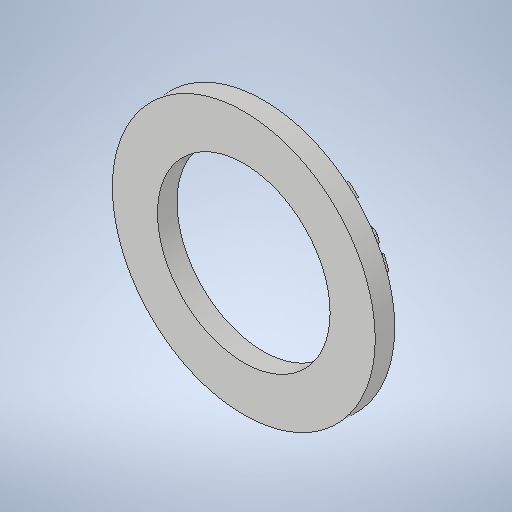
# Autodesk Inventor part: Fixierplatte_Innenring35mm
Saved by Autodesk Inventor 2025 (Build 290162000, 162)
## iProperties
Created: 2020-01-21
Part Number: Fixierplatte_Innenring35mm
Material: Generisch
Document SubType Name: Modeling
Designer: maxse
Density: 1 g/cm^3
Appearance: Vorgabe
Author: maxse
Autodesk Inventor part; units mm, degrees
(part 1 of 2)
ref_plane "YZ Plane" through (0, 0, 0) normal (1, 0, 0) x (0, 1, 0)
ref_plane "XZ Plane" through (0, 0, 0) normal (0, 1, 0) x (-1, 0, 0)
ref_plane "XY Plane" through (0, 0, 0) normal (0, 0, 1) x (1, 0, 0)
sketch "Skizze1" plane through (0, 0, 0) normal (0, 1, 0) x (-1, 0, 0)
  circle A0 centre (0, 0) radius 17.665
  circle A1 centre (0, 0) radius 26.9
  dimension "d0" = 35.33
  dimension "d1" = 53.8
  constraints: 2 centre point, 2 coincident
  measures "d0" diameter of A0
  measures "d1" diameter of A1
extrude "Extrusion1" add sketch "Skizze1" along normal blind 4
sketch "Skizze2" plane through (0, 4, 0) normal (0, 1, 0) x (1, 0, 0)
  circle A0 centre (0, 0) radius 19.096
  spline S0 degree 2 poles (20.5196, -9.7896) (20.1844, -9.6564) (19.6974, -9.2143) (19.5643, -8.9347) knots 0 0 0 1 2 2 2
  spline S1 degree 2 poles (19.5643, -8.9347) (19.4313, -8.6551) (19.4185, -7.9742) (19.5621, -7.6127) knots 0 0 0 1 2 2 2
  spline S2 degree 2 poles (19.5621, -7.6127) (19.6938, -7.2814) (20.098, -6.6921) (20.309, -6.5012) knots 0 0 0 1 2 2 2
  line L0 (20.309, -6.5012) -> (20.968, -6.7631)
  line L1 (20.968, -6.7631) -> (20.95, -6.8083)
  spline S3 degree 2 poles (20.95, -6.8083) (20.8689, -6.8589) (20.6271, -7.0724) (20.5025, -7.2103) knots 0 0 0 1 2 2 2
  spline S4 degree 2 poles (20.5025, -7.2103) (20.3652, -7.3694) (20.1724, -7.646) (20.0961, -7.838) knots 0 0 0 1 2 2 2
  spline S5 degree 2 poles (20.0961, -7.838) (20.0213, -8.0263) (20.0162, -8.4341) (20.1121, -8.6205) knots 0 0 0 1 2 2 2
  spline S6 degree 2 poles (20.1121, -8.6205) (20.2051, -8.7926) (20.5262, -9.0597) (20.7747, -9.1585) knots 0 0 0 1 2 2 2
  spline S7 degree 2 poles (20.7747, -9.1585) (21.0232, -9.2572) (21.3934, -9.2474) (21.5497, -9.1613) knots 0 0 0 1 2 2 2
  spline S8 degree 2 poles (21.5497, -9.1613) (21.7188, -9.0759) (21.9723, -8.7232) (22.0666, -8.4859) knots 0 0 0 1 2 2 2
  spline S9 degree 2 poles (22.0666, -8.4859) (22.1684, -8.2299) (22.2913, -7.6901) (22.3188, -7.5223) knots 0 0 0 1 2 2 2
  line L2 (22.3188, -7.5223) -> (24.7136, -8.474)
  line L3 (24.7136, -8.474) -> (23.7005, -11.0232)
  line L4 (23.7005, -11.0232) -> (23.1545, -10.8062)
  line L5 (23.1545, -10.8062) -> (23.9297, -8.8557)
  line L6 (23.9297, -8.8557) -> (22.6908, -8.3634)
  spline S10 degree 2 poles (22.6908, -8.3634) (22.661, -8.4824) (22.5855, -8.7052) (22.5496, -8.7956) knots 0 0 0 1 2 2 2
  spline S11 degree 2 poles (22.5496, -8.7956) (22.4074, -9.1533) (22.0947, -9.6002) (21.8317, -9.7573) knots 0 0 0 1 2 2 2
  spline S12 degree 2 poles (21.8317, -9.7573) (21.5672, -9.9182) (20.9413, -9.9572) (20.5196, -9.7896) knots 0 0 0 1 2 2 2
  spline S13 degree 2 poles (21.8528, -13.3779) (21.9489, -13.223) (22.0634, -12.8696) (22.0968, -12.6852) knots 0 0 0 1 2 2 2
  spline S14 degree 2 poles (22.0968, -12.6852) (22.1238, -12.5112) (22.126, -12.2312) (22.1201, -12.1178) knots 0 0 0 1 2 2 2
  line L7 (22.1201, -12.1178) -> (22.1414, -12.0834)
  line L8 (22.1414, -12.0834) -> (22.7438, -12.4574)
  spline S15 degree 2 poles (22.7438, -12.4574) (22.7282, -12.7053) (22.4946, -13.4425) (22.3172, -13.7283) knots 0 0 0 1 2 2 2
  spline S16 degree 2 poles (22.3172, -13.7283) (22.1377, -14.0174) (21.7535, -14.375) (21.5206, -14.4736) knots 0 0 0 1 2 2 2
  spline S17 degree 2 poles (21.5206, -14.4736) (21.2709, -14.5762) (20.7622, -14.5274) (20.5006, -14.365) knots 0 0 0 1 2 2 2
  spline S18 degree 2 poles (20.5006, -14.365) (20.1495, -14.147) (19.9058, -13.3565) (20.0378, -12.9902) knots 0 0 0 1 2 2 2
  line L9 (20.0378, -12.9902) -> (19.9965, -12.9646)
  spline S19 degree 2 poles (19.9965, -12.9646) (19.8856, -13.0817) (19.5715, -13.3111) (19.3664, -13.365) knots 0 0 0 1 2 2 2
  spline S20 degree 2 poles (19.3664, -13.365) (19.1647, -13.421) (18.6765, -13.3468) (18.3977, -13.1737) knots 0 0 0 1 2 2 2
  spline S21 degree 2 poles (18.3977, -13.1737) (18.112, -12.9963) (17.7485, -12.4987) (17.6737, -12.2043) knots 0 0 0 1 2 2 2
  spline S22 degree 2 poles (17.6737, -12.2043) (17.5964, -11.8987) (17.7237, -11.2481) (17.9311, -10.9142) knots 0 0 0 1 2 2 2
  spline S23 degree 2 poles (17.9311, -10.9142) (18.1298, -10.5941) (18.6737, -10.0638) (18.913, -9.9166) knots 0 0 0 1 2 2 2
  line L10 (18.913, -9.9166) -> (19.5154, -10.2906)
  line L11 (19.5154, -10.2906) -> (19.4897, -10.3319)
  spline S24 degree 2 poles (19.4897, -10.3319) (19.2478, -10.4297) (18.6306, -10.886) (18.4447, -11.1854) knots 0 0 0 1 2 2 2
  spline S25 degree 2 poles (18.4447, -11.1854) (18.3357, -11.361) (18.2278, -11.7805) (18.2825, -11.9766) knots 0 0 0 1 2 2 2
  spline S26 degree 2 poles (18.2825, -11.9766) (18.3393, -12.1693) (18.5675, -12.4779) (18.7981, -12.6211) knots 0 0 0 1 2 2 2
  spline S27 degree 2 poles (18.7981, -12.6211) (19.0287, -12.7643) (19.4116, -12.816) (19.5724, -12.7489) knots 0 0 0 1 2 2 2
  spline S28 degree 2 poles (19.5724, -12.7489) (19.7333, -12.6819) (20.0017, -12.3955) (20.1214, -12.2027) knots 0 0 0 1 2 2 2
  line L12 (20.1214, -12.2027) -> (20.271, -11.9617)
  line L13 (20.271, -11.9617) -> (20.7426, -12.2546)
  line L14 (20.7426, -12.2546) -> (20.6251, -12.4439)
  spline S29 degree 2 poles (20.6251, -12.4439) (20.3878, -12.826) (20.4535, -13.5345) (20.8012, -13.7503) knots 0 0 0 1 2 2 2
  spline S30 degree 2 poles (20.8012, -13.7503) (20.9629, -13.8508) (21.2705, -13.8701) (21.4014, -13.813) knots 0 0 0 1 2 2 2
  spline S31 degree 2 poles (21.4014, -13.813) (21.5399, -13.7512) (21.7609, -13.5259) (21.8528, -13.3779) knots 0 0 0 1 2 2 2
  line L15 (15.967, -13.7933) -> (16.4799, -13.1765)
  line L16 (16.4799, -13.1765) -> (17.2152, -13.7878)
  line L17 (17.2152, -13.7878) -> (16.7022, -14.4047)
  line L18 (16.7022, -14.4047) -> (15.967, -13.7933)
  spline S32 degree 2 poles (14.1579, -17.7888) (13.915, -17.5223) (13.6708, -16.9115) (13.6737, -16.6019) knots 0 0 0 1 2 2 2
  spline S33 degree 2 poles (13.6737, -16.6019) (13.6765, -16.2923) (13.9633, -15.6746) (14.2508, -15.4125) knots 0 0 0 1 2 2 2
  spline S34 degree 2 poles (14.2508, -15.4125) (14.5143, -15.1723) (15.1358, -14.8197) (15.4091, -14.7405) knots 0 0 0 1 2 2 2
  line L19 (15.4091, -14.7405) -> (15.8867, -15.2646)
  line L20 (15.8867, -15.2646) -> (15.8508, -15.2973)
  spline S35 degree 2 poles (15.8508, -15.2973) (15.7557, -15.3073) (15.4448, -15.3933) (15.2724, -15.4627) knots 0 0 0 1 2 2 2
  spline S36 degree 2 poles (15.2724, -15.4627) (15.0793, -15.5456) (14.7848, -15.7097) (14.6321, -15.8489) knots 0 0 0 1 2 2 2
  spline S37 degree 2 poles (14.6321, -15.8489) (14.4824, -15.9854) (14.2991, -16.3498) (14.3038, -16.5594) knots 0 0 0 1 2 2 2
  spline S38 degree 2 poles (14.3038, -16.5594) (14.3119, -16.7548) (14.4836, -17.1356) (14.6637, -17.3333) knots 0 0 0 1 2 2 2
  spline S39 degree 2 poles (14.6637, -17.3333) (14.8439, -17.5309) (15.181, -17.6842) (15.3592, -17.6752) knots 0 0 0 1 2 2 2
  spline S40 degree 2 poles (15.3592, -17.6752) (15.5486, -17.6725) (15.931, -17.4665) (16.1197, -17.2946) knots 0 0 0 1 2 2 2
  spline S41 degree 2 poles (16.1197, -17.2946) (16.3233, -17.109) (16.6703, -16.6776) (16.7685, -16.5387) knots 0 0 0 1 2 2 2
  line L21 (16.7685, -16.5387) -> (18.5044, -18.4433)
  line L22 (18.5044, -18.4433) -> (16.4771, -20.2912)
  line L23 (16.4771, -20.2912) -> (16.0813, -19.8569)
  line L24 (16.0813, -19.8569) -> (17.6325, -18.4431)
  line L25 (17.6325, -18.4431) -> (16.7345, -17.4579)
  spline S42 degree 2 poles (16.7345, -17.4579) (16.6556, -17.5517) (16.4901, -17.719) (16.4182, -17.7845) knots 0 0 0 1 2 2 2
  spline S43 degree 2 poles (16.4182, -17.7845) (16.1337, -18.0438) (15.6568, -18.3085) (15.3516, -18.3346) knots 0 0 0 1 2 2 2
  spline S44 degree 2 poles (15.3516, -18.3346) (15.0434, -18.3633) (14.4636, -18.1242) (14.1579, -17.7888) knots 0 0 0 1 2 2 2
  line L26 (8.7906, -19.2639) -> (9.8592, -21.1546)
  spline S45 degree 2 poles (9.8592, -21.1546) (9.9868, -21.3804) (10.2394, -21.745) (10.3556, -21.8189) knots 0 0 0 1 2 2 2
  spline S46 degree 2 poles (10.3556, -21.8189) (10.4779, -21.9034) (10.7568, -21.8947) (10.9438, -21.789) knots 0 0 0 1 2 2 2
  spline S47 degree 2 poles (10.9438, -21.789) (11.1131, -21.6933) (11.3835, -21.2659) (11.4765, -20.9527) knots 0 0 0 1 2 2 2
  spline S48 degree 2 poles (11.4765, -20.9527) (11.445, -20.9053) (11.3602, -20.7717) (11.3084, -20.68) knots 0 0 0 1 2 2 2
  line L27 (11.3084, -20.68) -> (10.0923, -18.5283)
  line L28 (10.0923, -18.5283) -> (10.6426, -18.2173)
  line L29 (10.6426, -18.2173) -> (11.7111, -20.108)
  spline S49 degree 2 poles (11.7111, -20.108) (11.8387, -20.3338) (12.0913, -20.6983) (12.2076, -20.7722) knots 0 0 0 1 2 2 2
  spline S50 degree 2 poles (12.2076, -20.7722) (12.3298, -20.8567) (12.6088, -20.848) (12.7957, -20.7424) knots 0 0 0 1 2 2 2
  spline S51 degree 2 poles (12.7957, -20.7424) (12.9721, -20.6427) (13.238, -20.1992) (13.3238, -19.9226) knots 0 0 0 1 2 2 2
  line L30 (13.3238, -19.9226) -> (11.9442, -17.4816)
  line L31 (11.9442, -17.4816) -> (12.4945, -17.1706)
  line L32 (12.4945, -17.1706) -> (14.3406, -20.4371)
  line L33 (14.3406, -20.4371) -> (13.7903, -20.7481)
  line L34 (13.7903, -20.7481) -> (13.5869, -20.3883)
  spline S52 degree 2 poles (13.5869, -20.3883) (13.4934, -20.7251) (13.2036, -21.2006) (12.9497, -21.3442) knots 0 0 0 1 2 2 2
  spline S53 degree 2 poles (12.9497, -21.3442) (12.6604, -21.5076) (12.0629, -21.4963) (11.777, -21.2622) knots 0 0 0 1 2 2 2
  spline S54 degree 2 poles (11.777, -21.2622) (11.6841, -21.6824) (11.3729, -22.2353) (11.0977, -22.3908) knots 0 0 0 1 2 2 2
  spline S55 degree 2 poles (11.0977, -22.3908) (10.8861, -22.5104) (10.4666, -22.5753) (10.2559, -22.4989) knots 0 0 0 1 2 2 2
  spline S56 degree 2 poles (10.2559, -22.4989) (10.0417, -22.4245) (9.6458, -22.0618) (9.4565, -21.7267) knots 0 0 0 1 2 2 2
  line L35 (9.4565, -21.7267) -> (8.2403, -19.5749)
  line L36 (8.2403, -19.5749) -> (8.7906, -19.2639)
  line L37 (3.2919, -20.9174) -> (3.8132, -23.0257)
  spline S57 degree 2 poles (3.8132, -23.0257) (3.8755, -23.2774) (4.0208, -23.6964) (4.1129, -23.7989) knots 0 0 0 1 2 2 2
  spline S58 degree 2 poles (4.1129, -23.7989) (4.2079, -23.9131) (4.479, -23.9797) (4.6875, -23.9281) knots 0 0 0 1 2 2 2
  spline S59 degree 2 poles (4.6875, -23.9281) (4.8763, -23.8814) (5.2516, -23.5424) (5.4252, -23.2657) knots 0 0 0 1 2 2 2
  spline S60 degree 2 poles (5.4252, -23.2657) (5.4077, -23.2116) (5.3619, -23.0601) (5.3366, -22.9579) knots 0 0 0 1 2 2 2
  line L38 (5.3366, -22.9579) -> (4.7433, -20.5585)
  line L39 (4.7433, -20.5585) -> (5.3569, -20.4068)
  line L40 (5.3569, -20.4068) -> (5.8782, -22.5151)
  spline S61 degree 2 poles (5.8782, -22.5151) (5.9405, -22.7668) (6.0858, -23.1858) (6.178, -23.2883) knots 0 0 0 1 2 2 2
  spline S62 degree 2 poles (6.178, -23.2883) (6.273, -23.4025) (6.544, -23.469) (6.7525, -23.4175) knots 0 0 0 1 2 2 2
  spline S63 degree 2 poles (6.7525, -23.4175) (6.9492, -23.3689) (7.3245, -23.0131) (7.4814, -22.7698) knots 0 0 0 1 2 2 2
  line L41 (7.4814, -22.7698) -> (6.8083, -20.0479)
  line L42 (6.8083, -20.0479) -> (7.422, -19.8962)
  line L43 (7.422, -19.8962) -> (8.3226, -23.5385)
  line L44 (8.3226, -23.5385) -> (7.709, -23.6902)
  line L45 (7.709, -23.6902) -> (7.6098, -23.289)
  spline S64 degree 2 poles (7.6098, -23.289) (7.4292, -23.5883) (7.0223, -23.9685) (6.7391, -24.0385) knots 0 0 0 1 2 2 2
  spline S65 degree 2 poles (6.7391, -24.0385) (6.4166, -24.1183) (5.8441, -23.9468) (5.6316, -23.6446) knots 0 0 0 1 2 2 2
  spline S66 degree 2 poles (5.6316, -23.6446) (5.4292, -24.0244) (4.9809, -24.4733) (4.6741, -24.5492) knots 0 0 0 1 2 2 2
  spline S67 degree 2 poles (4.6741, -24.5492) (4.4381, -24.6075) (4.0166, -24.5573) (3.8342, -24.4271) knots 0 0 0 1 2 2 2
  spline S68 degree 2 poles (3.8342, -24.4271) (3.6478, -24.2979) (3.364, -23.8422) (3.2716, -23.4685) knots 0 0 0 1 2 2 2
  line L46 (3.2716, -23.4685) -> (2.6783, -21.0691)
  line L47 (2.6783, -21.0691) -> (3.2919, -20.9174)
  spline S69 degree 2 poles (-1.4876, -20.975) (-0.9736, -21.0007) (-0.4242, -21.6163) (-0.4558, -22.2516) knots 0 0 0 1 2 2 2
  line L48 (-0.4558, -22.2516) -> (-0.5593, -24.3277)
  line L49 (-0.5593, -24.3277) -> (-0.1344, -24.3488)
  line L50 (-0.1344, -24.3488) -> (-0.1604, -24.8709)
  line L51 (-0.1604, -24.8709) -> (-0.5853, -24.8497)
  line L52 (-0.5853, -24.8497) -> (-0.639, -25.9262)
  line L53 (-0.639, -25.9262) -> (-1.2703, -25.8947)
  line L54 (-1.2703, -25.8947) -> (-1.2166, -24.8182)
  line L55 (-1.2166, -24.8182) -> (-2.3781, -24.7604)
  line L56 (-2.3781, -24.7604) -> (-2.3521, -24.2383)
  line L57 (-2.3521, -24.2383) -> (-1.1906, -24.2962)
  line L58 (-1.1906, -24.2962) -> (-1.1017, -22.5115)
  spline S70 degree 2 poles (-1.1017, -22.5115) (-1.0876, -22.2283) (-1.0923, -21.9157) (-1.1544, -21.7787) knots 0 0 0 1 2 2 2
  spline S71 degree 2 poles (-1.1544, -21.7787) (-1.2052, -21.6585) (-1.4543, -21.5284) (-1.6728, -21.5175) knots 0 0 0 1 2 2 2
  spline S72 degree 2 poles (-1.6728, -21.5175) (-1.8266, -21.5099) (-2.1186, -21.5886) (-2.1847, -21.6137) knots 0 0 0 1 2 2 2
  line L59 (-2.1847, -21.6137) -> (-2.2212, -21.6119)
  line L60 (-2.2212, -21.6119) -> (-2.1929, -21.0454)
  spline S73 degree 2 poles (-2.1929, -21.0454) (-2.0124, -21.0057) (-1.6454, -20.9672) (-1.4876, -20.975) knots 0 0 0 1 2 2 2
  spline S74 degree 2 poles (-6.0395, -22.2271) (-5.8581, -21.2965) (-4.7656, -20.4568) (-4.018, -20.6025) knots 0 0 0 1 2 2 2
  spline S75 degree 2 poles (-4.018, -20.6025) (-3.2504, -20.7521) (-2.5754, -21.9694) (-2.7506, -22.8682) knots 0 0 0 1 2 2 2
  spline S76 degree 2 poles (-2.7506, -22.8682) (-2.9304, -23.7909) (-4.0364, -24.6362) (-4.7761, -24.492) knots 0 0 0 1 2 2 2
  spline S77 degree 2 poles (-4.7761, -24.492) (-5.5238, -24.3463) (-6.2202, -23.1538) (-6.0395, -22.2271) knots 0 0 0 1 2 2 2
  spline S78 degree 2 poles (-5.3992, -22.3519) (-5.5388, -23.0678) (-5.1535, -23.8653) (-4.6722, -23.9591) knots 0 0 0 1 2 2 2
  spline S79 degree 2 poles (-4.6722, -23.9591) (-4.191, -24.0529) (-3.5304, -23.4593) (-3.3909, -22.7434) knots 0 0 0 1 2 2 2
  spline S80 degree 2 poles (-3.3909, -22.7434) (-3.2552, -22.0474) (-3.6406, -21.2292) (-4.1218, -21.1354) knots 0 0 0 1 2 2 2
  spline S81 degree 2 poles (-4.1218, -21.1354) (-4.5991, -21.0424) (-5.2613, -21.644) (-5.3992, -22.3519) knots 0 0 0 1 2 2 2
  spline S82 degree 2 poles (-11.4852, -22.9042) (-11.3227, -22.9869) (-10.9609, -23.0712) (-10.7744, -23.0889) knots 0 0 0 1 2 2 2
  spline S83 degree 2 poles (-10.7744, -23.0889) (-10.5987, -23.1011) (-10.3195, -23.0796) (-10.207, -23.0641) knots 0 0 0 1 2 2 2
  line L61 (-10.207, -23.0641) -> (-10.1709, -23.0825)
  line L62 (-10.1709, -23.0825) -> (-10.4928, -23.7144)
  spline S84 degree 2 poles (-10.4928, -23.7144) (-10.7411, -23.7197) (-11.4954, -23.5492) (-11.7951, -23.3966) knots 0 0 0 1 2 2 2
  spline S85 degree 2 poles (-11.7951, -23.3966) (-12.0984, -23.2421) (-12.4872, -22.8894) (-12.6051, -22.6657) knots 0 0 0 1 2 2 2
  spline S86 degree 2 poles (-12.6051, -22.6657) (-12.7283, -22.4255) (-12.7227, -21.9146) (-12.5829, -21.6402) knots 0 0 0 1 2 2 2
  spline S87 degree 2 poles (-12.5829, -21.6402) (-12.3953, -21.2719) (-11.6283, -20.9623) (-11.2521, -21.063) knots 0 0 0 1 2 2 2
  line L63 (-11.2521, -21.063) -> (-11.2301, -21.0197)
  spline S88 degree 2 poles (-11.2301, -21.0197) (-11.3562, -20.9191) (-11.6113, -20.6254) (-11.6823, -20.4256) knots 0 0 0 1 2 2 2
  spline S89 degree 2 poles (-11.6823, -20.4256) (-11.7551, -20.2293) (-11.7224, -19.7367) (-11.5735, -19.4442) knots 0 0 0 1 2 2 2
  spline S90 degree 2 poles (-11.5735, -19.4442) (-11.4208, -19.1445) (-10.9557, -18.7403) (-10.6686, -18.641) knots 0 0 0 1 2 2 2
  spline S91 degree 2 poles (-10.6686, -18.641) (-10.3707, -18.5381) (-9.7116, -18.6101) (-9.3614, -18.7885) knots 0 0 0 1 2 2 2
  spline S92 degree 2 poles (-9.3614, -18.7885) (-9.0256, -18.9595) (-8.4513, -19.4567) (-8.2845, -19.6826) knots 0 0 0 1 2 2 2
  line L64 (-8.2845, -19.6826) -> (-8.6063, -20.3145)
  line L65 (-8.6063, -20.3145) -> (-8.6496, -20.2924)
  spline S93 degree 2 poles (-8.6496, -20.2924) (-8.7675, -20.0596) (-9.2742, -19.4832) (-9.5883, -19.3232) knots 0 0 0 1 2 2 2
  spline S94 degree 2 poles (-9.5883, -19.3232) (-9.7724, -19.2294) (-10.1996, -19.1573) (-10.3904, -19.2284) knots 0 0 0 1 2 2 2
  spline S95 degree 2 poles (-10.3904, -19.2284) (-10.5775, -19.3013) (-10.8658, -19.5546) (-10.989, -19.7965) knots 0 0 0 1 2 2 2
  spline S96 degree 2 poles (-10.989, -19.7965) (-11.1122, -20.0384) (-11.1314, -20.4242) (-11.051, -20.5789) knots 0 0 0 1 2 2 2
  spline S97 degree 2 poles (-11.051, -20.5789) (-10.9706, -20.7335) (-10.6626, -20.9768) (-10.4604, -21.0798) knots 0 0 0 1 2 2 2
  line L66 (-10.4604, -21.0798) -> (-10.2077, -21.2085)
  line L67 (-10.2077, -21.2085) -> (-10.4596, -21.7032)
  line L68 (-10.4596, -21.7032) -> (-10.6582, -21.602)
  spline S98 degree 2 poles (-10.6582, -21.602) (-11.0589, -21.3979) (-11.7593, -21.5231) (-11.9451, -21.8878) knots 0 0 0 1 2 2 2
  spline S99 degree 2 poles (-11.9451, -21.8878) (-12.0315, -22.0575) (-12.0248, -22.3656) (-11.9569, -22.4911) knots 0 0 0 1 2 2 2
  spline S100 degree 2 poles (-11.9569, -22.4911) (-11.8836, -22.6239) (-11.6404, -22.8251) (-11.4852, -22.9042) knots 0 0 0 1 2 2 2
  spline S101 degree 2 poles (-14.9124, -17.1612) (-14.6946, -16.8738) (-14.1385, -16.5225) (-13.8336, -16.4689) knots 0 0 0 1 2 2 2
  spline S102 degree 2 poles (-13.8336, -16.4689) (-13.5286, -16.4153) (-12.869, -16.5848) (-12.559, -16.8197) knots 0 0 0 1 2 2 2
  spline S103 degree 2 poles (-12.559, -16.8197) (-12.2748, -17.0351) (-11.8148, -17.582) (-11.6872, -17.8362) knots 0 0 0 1 2 2 2
  line L69 (-11.6872, -17.8362) -> (-12.1155, -18.4014)
  line L70 (-12.1155, -18.4014) -> (-12.1543, -18.372)
  spline S104 degree 2 poles (-12.1543, -18.372) (-12.1814, -18.2803) (-12.3225, -17.9903) (-12.4222, -17.8334) knots 0 0 0 1 2 2 2
  spline S105 degree 2 poles (-12.4222, -17.8334) (-12.5389, -17.6586) (-12.7539, -17.399) (-12.9186, -17.2741) knots 0 0 0 1 2 2 2
  spline S106 degree 2 poles (-12.9186, -17.2741) (-13.0801, -17.1518) (-13.4718, -17.038) (-13.677, -17.0807) knots 0 0 0 1 2 2 2
  spline S107 degree 2 poles (-13.677, -17.0807) (-13.8677, -17.1243) (-14.2108, -17.3625) (-14.3724, -17.5756) knots 0 0 0 1 2 2 2
  spline S108 degree 2 poles (-14.3724, -17.5756) (-14.5339, -17.7887) (-14.6232, -18.1481) (-14.5819, -18.3217) knots 0 0 0 1 2 2 2
  spline S109 degree 2 poles (-14.5819, -18.3217) (-14.5448, -18.5075) (-14.2726, -18.846) (-14.0691, -19.0002) knots 0 0 0 1 2 2 2
  spline S110 degree 2 poles (-14.0691, -19.0002) (-13.8495, -19.1666) (-13.3622, -19.4292) (-13.2078, -19.5004) knots 0 0 0 1 2 2 2
  line L71 (-13.2078, -19.5004) -> (-14.7643, -21.5542)
  line L72 (-14.7643, -21.5542) -> (-16.9505, -19.8974)
  line L73 (-16.9505, -19.8974) -> (-16.5956, -19.4292)
  line L74 (-16.5956, -19.4292) -> (-14.9229, -20.6969)
  line L75 (-14.9229, -20.6969) -> (-14.1177, -19.6345)
  spline S111 degree 2 poles (-14.1177, -19.6345) (-14.2244, -19.5739) (-14.419, -19.4417) (-14.4965, -19.383) knots 0 0 0 1 2 2 2
  spline S112 degree 2 poles (-14.4965, -19.383) (-14.8033, -19.1505) (-15.1504, -18.7297) (-15.2316, -18.4344) knots 0 0 0 1 2 2 2
  spline S113 degree 2 poles (-15.2316, -18.4344) (-15.316, -18.1365) (-15.1865, -17.5229) (-14.9124, -17.1612) knots 0 0 0 1 2 2 2
  line L76 (-17.3405, -12.1524) -> (-19.0049, -13.5475)
  spline S114 degree 2 poles (-19.0049, -13.5475) (-19.2037, -13.7141) (-19.5161, -14.0288) (-19.5677, -14.1566) knots 0 0 0 1 2 2 2
  spline S115 degree 2 poles (-19.5677, -14.1566) (-19.6285, -14.2922) (-19.5691, -14.5649) (-19.4311, -14.7295) knots 0 0 0 1 2 2 2
  spline S116 degree 2 poles (-19.4311, -14.7295) (-19.3062, -14.8785) (-18.8367, -15.0666) (-18.5118, -15.1009) knots 0 0 0 1 2 2 2
  spline S117 degree 2 poles (-18.5118, -15.1009) (-18.471, -15.0614) (-18.3551, -14.9537) (-18.2743, -14.886) knots 0 0 0 1 2 2 2
  line L77 (-18.2743, -14.886) -> (-16.3801, -13.2983)
  line L78 (-16.3801, -13.2983) -> (-15.974, -13.7827)
  line L79 (-15.974, -13.7827) -> (-17.6385, -15.1778)
  spline S118 degree 2 poles (-17.6385, -15.1778) (-17.8372, -15.3444) (-18.1497, -15.6591) (-18.2012, -15.7869) knots 0 0 0 1 2 2 2
  spline S119 degree 2 poles (-18.2012, -15.7869) (-18.262, -15.9225) (-18.2026, -16.1952) (-18.0647, -16.3598) knots 0 0 0 1 2 2 2
  spline S120 degree 2 poles (-18.0647, -16.3598) (-17.9345, -16.5151) (-17.45, -16.6958) (-17.1625, -16.7297) knots 0 0 0 1 2 2 2
  line L80 (-17.1625, -16.7297) -> (-15.0136, -14.9286)
  line L81 (-15.0136, -14.9286) -> (-14.6076, -15.413)
  line L82 (-14.6076, -15.413) -> (-17.4831, -17.8232)
  line L83 (-17.4831, -17.8232) -> (-17.8891, -17.3388)
  line L84 (-17.8891, -17.3388) -> (-17.5724, -17.0733)
  spline S121 degree 2 poles (-17.5724, -17.0733) (-17.9206, -17.0426) (-18.441, -16.8444) (-18.6284, -16.6208) knots 0 0 0 1 2 2 2
  spline S122 degree 2 poles (-18.6284, -16.6208) (-18.8418, -16.3662) (-18.9395, -15.7766) (-18.7614, -15.4529) knots 0 0 0 1 2 2 2
  spline S123 degree 2 poles (-18.7614, -15.4529) (-19.1915, -15.438) (-19.7918, -15.2327) (-19.9948, -14.9905) knots 0 0 0 1 2 2 2
  spline S124 degree 2 poles (-19.9948, -14.9905) (-20.151, -14.8042) (-20.2912, -14.4035) (-20.2545, -14.1824) knots 0 0 0 1 2 2 2
  spline S125 degree 2 poles (-20.2545, -14.1824) (-20.2203, -13.9582) (-19.9358, -13.5029) (-19.6408, -13.2557) knots 0 0 0 1 2 2 2
  line L85 (-19.6408, -13.2557) -> (-17.7465, -11.668)
  line L86 (-17.7465, -11.668) -> (-17.3405, -12.1524)
  line L87 (-19.9679, -7.0468) -> (-21.9459, -7.9435)
  spline S126 degree 2 poles (-21.9459, -7.9435) (-22.1821, -8.0505) (-22.5677, -8.2697) (-22.6516, -8.379) knots 0 0 0 1 2 2 2
  spline S127 degree 2 poles (-22.6516, -8.379) (-22.7466, -8.4932) (-22.7627, -8.7719) (-22.674, -8.9675) knots 0 0 0 1 2 2 2
  spline S128 degree 2 poles (-22.674, -8.9675) (-22.5937, -9.1446) (-22.192, -9.4519) (-21.8883, -9.5722) knots 0 0 0 1 2 2 2
  spline S129 degree 2 poles (-21.8883, -9.5722) (-21.8383, -9.5451) (-21.6977, -9.4725) (-21.6018, -9.429) knots 0 0 0 1 2 2 2
  line L88 (-21.6018, -9.429) -> (-19.3506, -8.4086)
  line L89 (-19.3506, -8.4086) -> (-19.0897, -8.9843)
  line L90 (-19.0897, -8.9843) -> (-21.0677, -9.8809)
  spline S130 degree 2 poles (-21.0677, -9.8809) (-21.3039, -9.988) (-21.6895, -10.2072) (-21.7734, -10.3165) knots 0 0 0 1 2 2 2
  spline S131 degree 2 poles (-21.7734, -10.3165) (-21.8684, -10.4307) (-21.8845, -10.7094) (-21.7958, -10.905) knots 0 0 0 1 2 2 2
  spline S132 degree 2 poles (-21.7958, -10.905) (-21.7122, -11.0895) (-21.294, -11.3937) (-21.0262, -11.5037) knots 0 0 0 1 2 2 2
  line L91 (-21.0262, -11.5037) -> (-18.4724, -10.3461)
  line L92 (-18.4724, -10.3461) -> (-18.2114, -10.9218)
  line L93 (-18.2114, -10.9218) -> (-21.6288, -12.4708)
  line L94 (-21.6288, -12.4708) -> (-21.8897, -11.8951)
  line L95 (-21.8897, -11.8951) -> (-21.5133, -11.7245)
  spline S133 degree 2 poles (-21.5133, -11.7245) (-21.8405, -11.6014) (-22.2885, -11.2706) (-22.4089, -11.0049) knots 0 0 0 1 2 2 2
  spline S134 degree 2 poles (-22.4089, -11.0049) (-22.5461, -10.7023) (-22.4817, -10.1081) (-22.2233, -9.8442) knots 0 0 0 1 2 2 2
  spline S135 degree 2 poles (-22.2233, -9.8442) (-22.6336, -9.7143) (-23.1567, -9.3553) (-23.2871, -9.0674) knots 0 0 0 1 2 2 2
  spline S136 degree 2 poles (-23.2871, -9.0674) (-23.3875, -8.846) (-23.4149, -8.4224) (-23.3201, -8.2193) knots 0 0 0 1 2 2 2
  spline S137 degree 2 poles (-23.3201, -8.2193) (-23.227, -8.0125) (-22.8306, -7.6504) (-22.48, -7.4915) knots 0 0 0 1 2 2 2
  line L96 (-22.48, -7.4915) -> (-20.2288, -6.4711)
  line L97 (-20.2288, -6.4711) -> (-19.9679, -7.0468)
  constraints: 1 centre point, 1 coincident, 1 other
extrude "Extrusion2" add sketch "Skizze2" along normal blind 1 contours S0 S1 S2 L0 L1 S3 S4 S5 S6 S7 S8 S9 L2 L3 L4 L5 L6 S10 S11 S12 | S13 S14 L7 L8 S15 S16 S17 S18 L9 S19 S20 S21 S22 S23 L10 L11 S24 S25 S26 S27 S28 L12 L13 L14 S29 S30 S31 | L15 L16 L17 L18 | S32 S33 S34 L19 L20 S35 S36 S37 S38 S39 S40 S41 L21 L22 L23 L24 L25 S42 S43 S44 | L26 S45 S46 S47 S48 L27 L28 L29 S49 S50 S51 L30 L31 L32 L33 L34 S52 S53 S54 S55 S56 L35 L36 | L37 S57 S58 S59 S60 L38 L39 L40 S61 S62 S63 L41 L42 L43 L44 L45 S64 S65 S66 S67 S68 L46 L47 | S69 L48 L49 L50 L51 L52 L53 L54 L55 L56 L57 L58 S70 S71 S72 L59 L60 S73 | S74 S75 S76 S77 | S82 S83 L61 L62 S84 S85 S86 S87 L63 S88 S89 S90 S91 S92 L64 L65 S93 S94 S95 S96 S97 L66 L67 L68 S98 S99 S100 | S101 S102 S103 L69 L70 S104 S105 S106 S107 S108 S109 S110 L71 L72 L73 L74 L75 S111 S112 S113 | L76 S114 S115 S116 S117 L77 L78 L79 S118 S119 S120 L80 L81 L82 L83 L84 S121 S122 S123 S124 S125 L85 L86 | L87 S126 S127 S128 S129 L88 L89 L90 S130 S131 S132 L91 L92 L93 L94 L95 S133 S134 S135 S136 S137 L96 L97
sketch "Skizze3" plane through (0, 4, 0) normal (0, 1, 0) x (1, 0, 0)
  circle A0 centre (0, 0) radius 19.1572
  spline S0 degree 2 poles (20.9731, 5.7523) (21.195, 5.7998) (21.6282, 5.7271) (21.7971, 5.6153) knots 0 0 0 1 2 2 2
  spline S1 degree 2 poles (21.7971, 5.6153) (22.0098, 5.4752) (22.2927, 5.0339) (22.371, 4.6678) knots 0 0 0 1 2 2 2
  line L0 (22.371, 4.6678) -> (22.4535, 4.2822)
  line L1 (22.4535, 4.2822) -> (23.7293, 4.5551)
  line L2 (23.7293, 4.5551) -> (23.8266, 4.1002)
  line L3 (23.8266, 4.1002) -> (20.404, 3.3683)
  line L4 (20.404, 3.3683) -> (20.2201, 4.2281)
  spline S2 degree 2 poles (20.2201, 4.2281) (20.1549, 4.5332) (20.1634, 4.9817) (20.2421, 5.1697) knots 0 0 0 1 2 2 2
  spline S3 degree 2 poles (20.2421, 5.1697) (20.3315, 5.3889) (20.6874, 5.6913) (20.9731, 5.7523) knots 0 0 0 1 2 2 2
  spline S4 degree 2 poles (21.0884, 5.281) (20.9109, 5.2431) (20.6763, 5.0653) (20.6198, 4.9227) knots 0 0 0 1 2 2 2
  spline S5 degree 2 poles (20.6198, 4.9227) (20.5708, 4.7991) (20.5742, 4.4982) (20.6199, 4.2846) knots 0 0 0 1 2 2 2
  line L5 (20.6199, 4.2846) -> (20.7005, 3.9074)
  line L6 (20.7005, 3.9074) -> (22.0652, 4.1992)
  line L7 (22.0652, 4.1992) -> (21.9987, 4.5098)
  spline S6 degree 2 poles (21.9987, 4.5098) (21.9394, 4.7872) (21.7777, 5.1094) (21.6375, 5.1954) knots 0 0 0 1 2 2 2
  spline S7 degree 2 poles (21.6375, 5.1954) (21.5129, 5.2761) (21.2521, 5.316) (21.0884, 5.281) knots 0 0 0 1 2 2 2
  spline S8 degree 2 poles (22.5207, 7.9565) (22.5753, 7.9177) (22.7667, 7.7896) (22.8337, 7.7221) knots 0 0 0 1 2 2 2
  spline S9 degree 2 poles (22.8337, 7.7221) (22.9294, 7.6311) (23.0596, 7.444) (23.1216, 7.2554) knots 0 0 0 1 2 2 2
  spline S10 degree 2 poles (23.1216, 7.2554) (23.1721, 7.1019) (23.1476, 6.7862) (23.0771, 6.6466) knots 0 0 0 1 2 2 2
  spline S11 degree 2 poles (23.0771, 6.6466) (23.0075, 6.5132) (22.7456, 6.2927) (22.5786, 6.2378) knots 0 0 0 1 2 2 2
  spline S12 degree 2 poles (22.5786, 6.2378) (22.3199, 6.1527) (21.8817, 6.2504) (21.6986, 6.4529) knots 0 0 0 1 2 2 2
  spline S13 degree 2 poles (21.6986, 6.4529) (21.5325, 6.6312) (21.2719, 7.1784) (21.144, 7.5036) knots 0 0 0 1 2 2 2
  line L8 (21.144, 7.5036) -> (21.0631, 7.477)
  spline S14 degree 2 poles (21.0631, 7.477) (20.9177, 7.4291) (20.7664, 7.2809) (20.7418, 7.1832) knots 0 0 0 1 2 2 2
  spline S15 degree 2 poles (20.7418, 7.1832) (20.7172, 7.0855) (20.7611, 6.8432) (20.8019, 6.7192) knots 0 0 0 1 2 2 2
  spline S16 degree 2 poles (20.8019, 6.7192) (20.8497, 6.5737) (21.0653, 6.2087) (21.2136, 6.0395) knots 0 0 0 1 2 2 2
  line L9 (21.2136, 6.0395) -> (21.2215, 6.0153)
  line L10 (21.2215, 6.0153) -> (20.7931, 5.8744)
  spline S17 degree 2 poles (20.7931, 5.8744) (20.7227, 5.9796) (20.4992, 6.3868) (20.4292, 6.5996) knots 0 0 0 1 2 2 2
  spline S18 degree 2 poles (20.4292, 6.5996) (20.3441, 6.8583) (20.3088, 7.2378) (20.3678, 7.4125) knots 0 0 0 1 2 2 2
  spline S19 degree 2 poles (20.3678, 7.4125) (20.425, 7.5836) (20.7066, 7.8255) (20.941, 7.9026) knots 0 0 0 1 2 2 2
  line L11 (20.941, 7.9026) -> (22.6465, 8.4637)
  line L12 (22.6465, 8.4637) -> (22.7848, 8.0434)
  line L13 (22.7848, 8.0434) -> (22.5207, 7.9565)
  line L14 (22.1705, 7.8413) -> (21.4781, 7.6135)
  spline S20 degree 2 poles (21.4781, 7.6135) (21.5412, 7.4671) (21.7368, 7.0268) (21.8268, 6.8982) knots 0 0 0 1 2 2 2
  spline S21 degree 2 poles (21.8268, 6.8982) (21.933, 6.748) (22.2176, 6.5998) (22.4062, 6.6618) knots 0 0 0 1 2 2 2
  spline S22 degree 2 poles (22.4062, 6.6618) (22.6218, 6.7327) (22.7602, 7.047) (22.684, 7.2787) knots 0 0 0 1 2 2 2
  spline S23 degree 2 poles (22.684, 7.2787) (22.6193, 7.4754) (22.3432, 7.7428) (22.1705, 7.8413) knots 0 0 0 1 2 2 2
  line L15 (19.882, 9.4667) -> (19.8909, 9.4458)
  spline S24 degree 2 poles (19.8909, 9.4458) (19.8981, 9.3933) (19.9366, 9.2894) (19.9668, 9.2191) knots 0 0 0 1 2 2 2
  spline S25 degree 2 poles (19.9668, 9.2191) (20.0374, 9.0549) (20.3196, 8.7934) (20.523, 8.708) knots 0 0 0 1 2 2 2
  line L16 (20.523, 8.708) -> (22.235, 9.4439)
  line L17 (22.235, 9.4439) -> (22.4097, 9.0374)
  line L18 (22.4097, 9.0374) -> (19.9968, 8.0002)
  line L19 (19.9968, 8.0002) -> (19.8221, 8.4067)
  line L20 (19.8221, 8.4067) -> (20.1817, 8.5612)
  spline S26 degree 2 poles (20.1817, 8.5612) (19.8884, 8.6976) (19.5846, 8.9591) (19.5174, 9.1154) knots 0 0 0 1 2 2 2
  spline S27 degree 2 poles (19.5174, 9.1154) (19.4905, 9.178) (19.4688, 9.2427) (19.4599, 9.2852) knots 0 0 0 1 2 2 2
  line L21 (19.4599, 9.2852) -> (19.882, 9.4667)
  line L22 (21.4966, 11.0234) -> (21.6949, 10.6278)
  line L23 (21.6949, 10.6278) -> (19.347, 9.4508)
  line L24 (19.347, 9.4508) -> (19.1487, 9.8464)
  line L25 (19.1487, 9.8464) -> (21.4966, 11.0234)
  line L26 (18.7442, 9.6785) -> (18.9692, 9.2297)
  line L27 (18.9692, 9.2297) -> (18.5585, 9.0238)
  line L28 (18.5585, 9.0238) -> (18.3335, 9.4726)
  line L29 (18.3335, 9.4726) -> (18.7442, 9.6785)
  spline S28 degree 2 poles (20.8964, 12.2447) (21.0301, 12.0174) (21.1395, 11.5519) (21.1473, 11.3821) knots 0 0 0 1 2 2 2
  line L30 (21.1473, 11.3821) -> (20.7195, 11.1303)
  line L31 (20.7195, 11.1303) -> (20.708, 11.1499)
  spline S29 degree 2 poles (20.708, 11.1499) (20.7183, 11.2218) (20.7336, 11.4085) (20.7202, 11.5487) knots 0 0 0 1 2 2 2
  spline S30 degree 2 poles (20.7202, 11.5487) (20.7105, 11.6713) (20.6409, 11.9463) (20.5675, 12.071) knots 0 0 0 1 2 2 2
  spline S31 degree 2 poles (20.5675, 12.071) (20.5143, 12.1614) (20.3505, 12.3447) (20.2875, 12.3735) knots 0 0 0 1 2 2 2
  spline S32 degree 2 poles (20.2875, 12.3735) (20.1993, 12.4171) (20.0568, 12.4188) (19.9493, 12.3555) knots 0 0 0 1 2 2 2
  spline S33 degree 2 poles (19.9493, 12.3555) (19.8148, 12.2764) (19.7618, 12.0477) (19.8261, 11.8321) knots 0 0 0 1 2 2 2
  spline S34 degree 2 poles (19.8261, 11.8321) (19.8521, 11.7487) (19.9413, 11.4853) (19.9734, 11.3693) knots 0 0 0 1 2 2 2
  spline S35 degree 2 poles (19.9734, 11.3693) (20.0501, 11.0655) (19.8753, 10.6468) (19.6528, 10.5159) knots 0 0 0 1 2 2 2
  spline S36 degree 2 poles (19.6528, 10.5159) (19.3448, 10.3346) (18.6892, 10.5708) (18.4648, 10.9522) knots 0 0 0 1 2 2 2
  spline S37 degree 2 poles (18.4648, 10.9522) (18.354, 11.1404) (18.2225, 11.5764) (18.2172, 11.7477) knots 0 0 0 1 2 2 2
  line L32 (18.2172, 11.7477) -> (18.6254, 11.9879)
  line L33 (18.6254, 11.9879) -> (18.6369, 11.9683)
  spline S38 degree 2 poles (18.6369, 11.9683) (18.6059, 11.7526) (18.6814, 11.3166) (18.7893, 11.1333) knots 0 0 0 1 2 2 2
  spline S39 degree 2 poles (18.7893, 11.1333) (18.9001, 10.945) (19.2114, 10.7794) (19.3703, 10.8729) knots 0 0 0 1 2 2 2
  spline S40 degree 2 poles (19.3703, 10.8729) (19.5146, 10.9578) (19.5633, 11.1938) (19.5066, 11.3908) knots 0 0 0 1 2 2 2
  spline S41 degree 2 poles (19.5066, 11.3908) (19.4797, 11.4868) (19.4, 11.7229) (19.3593, 11.8537) knots 0 0 0 1 2 2 2
  spline S42 degree 2 poles (19.3593, 11.8537) (19.2761, 12.1404) (19.4174, 12.5658) (19.6692, 12.7139) knots 0 0 0 1 2 2 2
  spline S43 degree 2 poles (19.6692, 12.7139) (19.8159, 12.8003) (20.1426, 12.8378) (20.3041, 12.7815) knots 0 0 0 1 2 2 2
  spline S44 degree 2 poles (20.3041, 12.7815) (20.4748, 12.7207) (20.7597, 12.477) (20.8964, 12.2447) knots 0 0 0 1 2 2 2
  line L34 (17.9093, 16.2552) -> (19.197, 14.6886)
  line L35 (19.197, 14.6886) -> (16.4932, 12.4661)
  line L36 (16.4932, 12.4661) -> (16.1978, 12.8255)
  line L37 (16.1978, 12.8255) -> (18.5818, 14.785)
  line L38 (18.5818, 14.785) -> (17.5894, 15.9923)
  line L39 (17.5894, 15.9923) -> (17.9093, 16.2552)
  spline S45 degree 2 poles (15.2199, 17.0757) (15.6863, 17.5479) (16.6486, 17.6139) (17.0279, 17.2392) knots 0 0 0 1 2 2 2
  spline S46 degree 2 poles (17.0279, 17.2392) (17.4174, 16.8545) (17.3391, 15.8833) (16.8886, 15.4272) knots 0 0 0 1 2 2 2
  spline S47 degree 2 poles (16.8886, 15.4272) (16.4261, 14.9591) (15.4538, 14.895) (15.0785, 15.2658) knots 0 0 0 1 2 2 2
  spline S48 degree 2 poles (15.0785, 15.2658) (14.6992, 15.6405) (14.7554, 16.6056) (15.2199, 17.0757) knots 0 0 0 1 2 2 2
  spline S49 degree 2 poles (15.5447, 16.7548) (15.186, 16.3916) (15.1015, 15.7773) (15.3456, 15.5362) knots 0 0 0 1 2 2 2
  spline S50 degree 2 poles (15.3456, 15.5362) (15.5898, 15.295) (16.2049, 15.385) (16.5637, 15.7482) knots 0 0 0 1 2 2 2
  spline S51 degree 2 poles (16.5637, 15.7482) (16.9125, 16.1013) (17.005, 16.7276) (16.7608, 16.9688) knots 0 0 0 1 2 2 2
  spline S52 degree 2 poles (16.7608, 16.9688) (16.5187, 17.208) (15.8996, 17.1139) (15.5447, 16.7548) knots 0 0 0 1 2 2 2
  line L40 (14.2151, 19.5582) -> (14.5618, 19.2833)
  line L41 (14.5618, 19.2833) -> (14.3962, 19.0744)
  spline S53 degree 2 poles (14.3962, 19.0744) (14.5291, 19.0776) (14.7174, 19.0732) (14.8273, 19.0475) knots 0 0 0 1 2 2 2
  spline S54 degree 2 poles (14.8273, 19.0475) (14.9289, 19.0249) (15.1166, 18.9376) (15.2211, 18.8548) knots 0 0 0 1 2 2 2
  spline S55 degree 2 poles (15.2211, 18.8548) (15.39, 18.7209) (15.5635, 18.3554) (15.5561, 18.1405) knots 0 0 0 1 2 2 2
  spline S56 degree 2 poles (15.5561, 18.1405) (15.5486, 17.9256) (15.3426, 17.4374) (15.1365, 17.1774) knots 0 0 0 1 2 2 2
  spline S57 degree 2 poles (15.1365, 17.1774) (14.9215, 16.9062) (14.4679, 16.6216) (14.2276, 16.5696) knots 0 0 0 1 2 2 2
  spline S58 degree 2 poles (14.2276, 16.5696) (14.0085, 16.5261) (13.5691, 16.6246) (13.3935, 16.7638) knots 0 0 0 1 2 2 2
  spline S59 degree 2 poles (13.3935, 16.7638) (13.2401, 16.8854) (13.0658, 17.1358) (12.9955, 17.3073) knots 0 0 0 1 2 2 2
  line L42 (12.9955, 17.3073) -> (12.2907, 16.4183)
  line L43 (12.2907, 16.4183) -> (11.944, 16.6931)
  line L44 (11.944, 16.6931) -> (14.2151, 19.5582)
  line L45 (14.1654, 18.7832) -> (13.2228, 17.5941)
  spline S60 degree 2 poles (13.2228, 17.5941) (13.3024, 17.4296) (13.4699, 17.2209) (13.5877, 17.1275) knots 0 0 0 1 2 2 2
  spline S61 degree 2 poles (13.5877, 17.1275) (13.8544, 16.9161) (14.4738, 17.0765) (14.7733, 17.4544) knots 0 0 0 1 2 2 2
  spline S62 degree 2 poles (14.7733, 17.4544) (15.0623, 17.8189) (15.1359, 18.3867) (14.8803, 18.5893) knots 0 0 0 1 2 2 2
  spline S63 degree 2 poles (14.8803, 18.5893) (14.7447, 18.6968) (14.3705, 18.7908) (14.1654, 18.7832) knots 0 0 0 1 2 2 2
  line L46 (11.3396, 18.8765) -> (11.3586, 18.8641)
  spline S64 degree 2 poles (11.3586, 18.8641) (11.3936, 18.8243) (11.483, 18.759) (11.5471, 18.7171) knots 0 0 0 1 2 2 2
  spline S65 degree 2 poles (11.5471, 18.7171) (11.6967, 18.6192) (12.0764, 18.5572) (12.2931, 18.5984) knots 0 0 0 1 2 2 2
  line L47 (12.2931, 18.5984) -> (13.3133, 20.1578)
  line L48 (13.3133, 20.1578) -> (13.6836, 19.9156)
  line L49 (13.6836, 19.9156) -> (12.2457, 17.7177)
  line L50 (12.2457, 17.7177) -> (11.8754, 17.96)
  line L51 (11.8754, 17.96) -> (12.0897, 18.2875)
  spline S66 degree 2 poles (12.0897, 18.2875) (11.77, 18.2391) (11.3723, 18.2892) (11.2299, 18.3823) knots 0 0 0 1 2 2 2
  spline S67 degree 2 poles (11.2299, 18.3823) (11.1729, 18.4196) (11.119, 18.4616) (11.0881, 18.492) knots 0 0 0 1 2 2 2
  line L52 (11.0881, 18.492) -> (11.3396, 18.8765)
  spline S68 degree 2 poles (9.7041, 20.7136) (10.0162, 21.2994) (10.9194, 21.6377) (11.3901, 21.3871) knots 0 0 0 1 2 2 2
  spline S69 degree 2 poles (11.3901, 21.3871) (11.8732, 21.1297) (12.0758, 20.1767) (11.7744, 19.6109) knots 0 0 0 1 2 2 2
  spline S70 degree 2 poles (11.7744, 19.6109) (11.4651, 19.0301) (10.5516, 18.6908) (10.086, 18.9388) knots 0 0 0 1 2 2 2
  spline S71 degree 2 poles (10.086, 18.9388) (9.6154, 19.1895) (9.3935, 20.1303) (9.7041, 20.7136) knots 0 0 0 1 2 2 2
  spline S72 degree 2 poles (10.1072, 20.4989) (9.8672, 20.0483) (9.9618, 19.4356) (10.2647, 19.2742) knots 0 0 0 1 2 2 2
  spline S73 degree 2 poles (10.2647, 19.2742) (10.5676, 19.1129) (11.1314, 19.375) (11.3714, 19.8256) knots 0 0 0 1 2 2 2
  spline S74 degree 2 poles (11.3714, 19.8256) (11.6047, 20.2637) (11.5143, 20.8903) (11.2114, 21.0516) knots 0 0 0 1 2 2 2
  spline S75 degree 2 poles (11.2114, 21.0516) (10.911, 21.2116) (10.3445, 20.9445) (10.1072, 20.4989) knots 0 0 0 1 2 2 2
  line L53 (7.9921, 22.8206) -> (8.403, 22.6566)
  line L54 (8.403, 22.6566) -> (7.8476, 21.2658)
  spline S76 degree 2 poles (7.8476, 21.2658) (7.7803, 21.0972) (7.6962, 20.7948) (7.7089, 20.689) knots 0 0 0 1 2 2 2
  spline S77 degree 2 poles (7.7089, 20.689) (7.7221, 20.5768) (7.8655, 20.4157) (8.0182, 20.3547) knots 0 0 0 1 2 2 2
  spline S78 degree 2 poles (8.0182, 20.3547) (8.171, 20.2937) (8.5602, 20.3276) (8.7682, 20.3973) knots 0 0 0 1 2 2 2
  line L55 (8.7682, 20.3973) -> (9.4961, 22.22)
  line L56 (9.4961, 22.22) -> (9.907, 22.0559)
  line L57 (9.907, 22.0559) -> (8.933, 19.6168)
  line L58 (8.933, 19.6168) -> (8.5221, 19.7809)
  line L59 (8.5221, 19.7809) -> (8.6304, 20.0522)
  spline S79 degree 2 poles (8.6304, 20.0522) (8.3798, 19.9599) (7.9548, 19.928) (7.7546, 20.008) knots 0 0 0 1 2 2 2
  spline S80 degree 2 poles (7.7546, 20.008) (7.3963, 20.151) (7.18, 20.7872) (7.3599, 21.2376) knots 0 0 0 1 2 2 2
  line L60 (7.3599, 21.2376) -> (7.9921, 22.8206)
  spline S81 degree 2 poles (4.744, 23.762) (5.0471, 23.7015) (5.4661, 23.4531) (5.593, 23.2629) knots 0 0 0 1 2 2 2
  spline S82 degree 2 poles (5.593, 23.2629) (5.7383, 23.0488) (5.7857, 22.5187) (5.7125, 22.1515) knots 0 0 0 1 2 2 2
  line L61 (5.7125, 22.1515) -> (5.285, 20.0098)
  line L62 (5.285, 20.0098) -> (4.8289, 20.1009)
  line L63 (4.8289, 20.1009) -> (5.2563, 22.2426)
  spline S83 degree 2 poles (5.2563, 22.2426) (5.3041, 22.4818) (5.3073, 22.8166) (5.2471, 22.9646) knots 0 0 0 1 2 2 2
  spline S84 degree 2 poles (5.2471, 22.9646) (5.1831, 23.122) (4.8943, 23.3271) (4.6662, 23.3726) knots 0 0 0 1 2 2 2
  spline S85 degree 2 poles (4.6662, 23.3726) (4.4521, 23.4154) (4.09, 23.3401) (3.9704, 23.2194) knots 0 0 0 1 2 2 2
  spline S86 degree 2 poles (3.9704, 23.2194) (3.8581, 23.1059) (3.7331, 22.7982) (3.687, 22.5674) knots 0 0 0 1 2 2 2
  line L64 (3.687, 22.5674) -> (3.2573, 20.4145)
  line L65 (3.2573, 20.4145) -> (2.8012, 20.5056)
  line L66 (2.8012, 20.5056) -> (3.2286, 22.6473)
  spline S87 degree 2 poles (3.2286, 22.6473) (3.3002, 23.0061) (3.547, 23.489) (3.7656, 23.6276) knots 0 0 0 1 2 2 2
  spline S88 degree 2 poles (3.7656, 23.6276) (3.9619, 23.7562) (4.4269, 23.8253) (4.744, 23.762) knots 0 0 0 1 2 2 2
  line L67 (0.8028, 24.1663) -> (1.244, 24.1326)
  line L68 (1.244, 24.1326) -> (1.1299, 22.6394)
  spline S89 degree 2 poles (1.1299, 22.6394) (1.116, 22.4584) (1.1262, 22.1447) (1.17, 22.0475) knots 0 0 0 1 2 2 2
  spline S90 degree 2 poles (1.17, 22.0475) (1.2162, 21.9444) (1.4011, 21.8335) (1.5651, 21.821) knots 0 0 0 1 2 2 2
  spline S91 degree 2 poles (1.5651, 21.821) (1.7292, 21.8085) (2.0904, 21.9572) (2.2681, 22.0859) knots 0 0 0 1 2 2 2
  line L69 (2.2681, 22.0859) -> (2.4176, 24.0429)
  line L70 (2.4176, 24.0429) -> (2.8588, 24.0092)
  line L71 (2.8588, 24.0092) -> (2.6587, 21.3904)
  line L72 (2.6587, 21.3904) -> (2.2175, 21.4241)
  line L73 (2.2175, 21.4241) -> (2.2398, 21.7154)
  spline S92 degree 2 poles (2.2398, 21.7154) (2.0282, 21.5524) (1.6321, 21.3949) (1.4172, 21.4113) knots 0 0 0 1 2 2 2
  spline S93 degree 2 poles (1.4172, 21.4113) (1.0326, 21.4407) (0.636, 21.983) (0.6729, 22.4666) knots 0 0 0 1 2 2 2
  line L74 (0.6729, 22.4666) -> (0.8028, 24.1663)
  line L75 (-0.2691, 24.1567) -> (0.1734, 24.1576)
  line L76 (0.1734, 24.1576) -> (0.1786, 21.5312)
  line L77 (0.1786, 21.5312) -> (-0.2639, 21.5303)
  line L78 (-0.2639, 21.5303) -> (-0.2691, 24.1567)
  line L79 (-0.2942, 21.0935) -> (0.2078, 21.0945)
  line L80 (0.2078, 21.0945) -> (0.2087, 20.635)
  line L81 (0.2087, 20.635) -> (-0.2933, 20.634)
  line L82 (-0.2933, 20.634) -> (-0.2942, 21.0935)
  line L83 (-2.7796, 21.3834) -> (-1.9875, 24.0761)
  line L84 (-1.9875, 24.0761) -> (-1.5915, 24.1056)
  line L85 (-1.5915, 24.1056) -> (-0.4178, 21.5593)
  line L86 (-0.4178, 21.5593) -> (-0.8958, 21.5237)
  line L87 (-0.8958, 21.5237) -> (-1.7616, 23.4871)
  line L88 (-1.7616, 23.4871) -> (-2.3214, 21.4176)
  line L89 (-2.3214, 21.4176) -> (-2.7796, 21.3834)
  spline S94 degree 2 poles (-4.4377, 23.8075) (-3.8178, 23.9179) (-3.0126, 23.344) (-2.8982, 22.7017) knots 0 0 0 1 2 2 2
  spline S95 degree 2 poles (-2.8982, 22.7017) (-2.7858, 22.0707) (-3.3143, 21.2044) (-3.8476, 21.1094) knots 0 0 0 1 2 2 2
  spline S96 degree 2 poles (-3.8476, 21.1094) (-4.0878, 21.0667) (-4.484, 21.1401) (-4.6472, 21.2638) knots 0 0 0 1 2 2 2
  spline S97 degree 2 poles (-4.6472, 21.2638) (-4.8132, 21.3869) (-5.0373, 21.7878) (-5.0925, 22.0977) knots 0 0 0 1 2 2 2
  line L90 (-5.0925, 22.0977) -> (-5.1348, 22.3351)
  line L91 (-5.1348, 22.3351) -> (-3.3449, 22.6539)
  spline S98 degree 2 poles (-3.3449, 22.6539) (-3.4249, 23.1034) (-3.9623, 23.5004) (-4.3644, 23.4287) knots 0 0 0 1 2 2 2
  spline S99 degree 2 poles (-4.3644, 23.4287) (-4.5069, 23.4034) (-4.7719, 23.2899) (-4.8746, 23.2198) knots 0 0 0 1 2 2 2
  spline S100 degree 2 poles (-4.8746, 23.2198) (-4.9819, 23.143) (-5.1265, 23.0164) (-5.1716, 22.9623) knots 0 0 0 1 2 2 2
  line L92 (-5.1716, 22.9623) -> (-5.1967, 22.9578)
  line L93 (-5.1967, 22.9578) -> (-5.2813, 23.4325)
  spline S101 degree 2 poles (-5.2813, 23.4325) (-5.2113, 23.4767) (-4.9983, 23.6068) (-4.9134, 23.6479) knots 0 0 0 1 2 2 2
  spline S102 degree 2 poles (-4.9134, 23.6479) (-4.7942, 23.7066) (-4.594, 23.7797) (-4.4377, 23.8075) knots 0 0 0 1 2 2 2
  spline S103 degree 2 poles (-4.6511, 22.0784) (-4.6142, 21.9034) (-4.4959, 21.6595) (-4.4106, 21.5854) knots 0 0 0 1 2 2 2
  spline S104 degree 2 poles (-4.4106, 21.5854) (-4.3178, 21.501) (-4.0621, 21.44) (-3.8862, 21.4713) knots 0 0 0 1 2 2 2
  spline S105 degree 2 poles (-3.8862, 21.4713) (-3.713, 21.5022) (-3.4885, 21.6488) (-3.4059, 21.7672) knots 0 0 0 1 2 2 2
  spline S106 degree 2 poles (-3.4059, 21.7672) (-3.3266, 21.8879) (-3.2703, 22.1543) (-3.2857, 22.3216) knots 0 0 0 1 2 2 2
  line L94 (-3.2857, 22.3216) -> (-4.6511, 22.0784)
  line L95 (-6.5694, 21.0179) -> (-6.5475, 21.0239)
  spline S107 degree 2 poles (-6.5475, 21.0239) (-6.4945, 21.0235) (-6.3863, 21.047) (-6.3123, 21.067) knots 0 0 0 1 2 2 2
  spline S108 degree 2 poles (-6.3123, 21.067) (-6.1399, 21.1137) (-5.8412, 21.3563) (-5.7279, 21.5456) knots 0 0 0 1 2 2 2
  line L96 (-5.7279, 21.5456) -> (-6.2152, 23.3442)
  line L97 (-6.2152, 23.3442) -> (-5.7881, 23.4599)
  line L98 (-5.7881, 23.4599) -> (-5.1014, 20.9249)
  line L99 (-5.1014, 20.9249) -> (-5.5284, 20.8092)
  line L100 (-5.5284, 20.8092) -> (-5.6308, 21.187)
  spline S109 degree 2 poles (-5.6308, 21.187) (-5.8071, 20.9159) (-6.1088, 20.652) (-6.2731, 20.6075) knots 0 0 0 1 2 2 2
  spline S110 degree 2 poles (-6.2731, 20.6075) (-6.3388, 20.5897) (-6.406, 20.5774) (-6.4493, 20.5744) knots 0 0 0 1 2 2 2
  line L101 (-6.4493, 20.5744) -> (-6.5694, 21.0179)
  spline S111 degree 2 poles (-8.1467, 22.8084) (-7.8984, 22.8976) (-7.4207, 22.9185) (-7.2524, 22.8946) knots 0 0 0 1 2 2 2
  line L102 (-7.2524, 22.8946) -> (-7.0846, 22.4275)
  line L103 (-7.0846, 22.4275) -> (-7.106, 22.4198)
  spline S112 degree 2 poles (-7.106, 22.4198) (-7.1747, 22.4433) (-7.3553, 22.493) (-7.4955, 22.5059) knots 0 0 0 1 2 2 2
  spline S113 degree 2 poles (-7.4955, 22.5059) (-7.6178, 22.5192) (-7.9009, 22.5019) (-8.0371, 22.453) knots 0 0 0 1 2 2 2
  spline S114 degree 2 poles (-8.0371, 22.453) (-8.1358, 22.4175) (-8.3464, 22.2906) (-8.3864, 22.2341) knots 0 0 0 1 2 2 2
  spline S115 degree 2 poles (-8.3864, 22.2341) (-8.4456, 22.1555) (-8.4738, 22.0158) (-8.4316, 21.8984) knots 0 0 0 1 2 2 2
  spline S116 degree 2 poles (-8.4316, 21.8984) (-8.3788, 21.7516) (-8.164, 21.657) (-7.9403, 21.6801) knots 0 0 0 1 2 2 2
  spline S117 degree 2 poles (-7.9403, 21.6801) (-7.8535, 21.6902) (-7.578, 21.7288) (-7.458, 21.7388) knots 0 0 0 1 2 2 2
  spline S118 degree 2 poles (-7.458, 21.7388) (-7.1454, 21.7577) (-6.7664, 21.508) (-6.6791, 21.2651) knots 0 0 0 1 2 2 2
  spline S119 degree 2 poles (-6.6791, 21.2651) (-6.5583, 20.9288) (-6.9123, 20.3285) (-7.3287, 20.1789) knots 0 0 0 1 2 2 2
  spline S120 degree 2 poles (-7.3287, 20.1789) (-7.5342, 20.1051) (-7.9871, 20.0569) (-8.1563, 20.0835) knots 0 0 0 1 2 2 2
  line L104 (-8.1563, 20.0835) -> (-8.3165, 20.5293)
  line L105 (-8.3165, 20.5293) -> (-8.2951, 20.537)
  spline S121 degree 2 poles (-8.2951, 20.537) (-8.0889, 20.4664) (-7.6465, 20.4596) (-7.4463, 20.5315) knots 0 0 0 1 2 2 2
  spline S122 degree 2 poles (-7.4463, 20.5315) (-7.2407, 20.6053) (-7.0201, 20.8804) (-7.0825, 21.054) knots 0 0 0 1 2 2 2
  spline S123 degree 2 poles (-7.0825, 21.054) (-7.139, 21.2114) (-7.3618, 21.3032) (-7.566, 21.2841) knots 0 0 0 1 2 2 2
  spline S124 degree 2 poles (-7.566, 21.2841) (-7.6653, 21.2755) (-7.9122, 21.2411) (-8.0482, 21.2254) knots 0 0 0 1 2 2 2
  spline S125 degree 2 poles (-8.0482, 21.2254) (-8.3454, 21.197) (-8.7371, 21.4149) (-8.8358, 21.6899) knots 0 0 0 1 2 2 2
  spline S126 degree 2 poles (-8.8358, 21.6899) (-8.8934, 21.85) (-8.8696, 22.178) (-8.7842, 22.3262) knots 0 0 0 1 2 2 2
  spline S127 degree 2 poles (-8.7842, 22.3262) (-8.6927, 22.4827) (-8.4003, 22.7173) (-8.1467, 22.8084) knots 0 0 0 1 2 2 2
  line L106 (-9.8775, 22.0467) -> (-9.4721, 22.2239)
  line L107 (-9.4721, 22.2239) -> (-8.4202, 19.8173)
  line L108 (-8.4202, 19.8173) -> (-8.8257, 19.6401)
  line L109 (-8.8257, 19.6401) -> (-9.8775, 22.0467)
  line L110 (-8.6793, 19.2273) -> (-8.2193, 19.4284)
  line L111 (-8.2193, 19.4284) -> (-8.0353, 19.0074)
  line L112 (-8.0353, 19.0074) -> (-8.4953, 18.8063)
  line L113 (-8.4953, 18.8063) -> (-8.6793, 19.2273)
  spline S128 degree 2 poles (-11.1998, 21.4639) (-10.8783, 21.6265) (-10.3308, 21.4425) (-10.1299, 21.0451) knots 0 0 0 1 2 2 2
  line L114 (-10.1299, 21.0451) -> (-9.4733, 19.7467)
  line L115 (-9.4733, 19.7467) -> (-9.2075, 19.881)
  line L116 (-9.2075, 19.881) -> (-9.0424, 19.5545)
  line L117 (-9.0424, 19.5545) -> (-9.3082, 19.4201)
  line L118 (-9.3082, 19.4201) -> (-8.9677, 18.7469)
  line L119 (-8.9677, 18.7469) -> (-9.3626, 18.5472)
  line L120 (-9.3626, 18.5472) -> (-9.703, 19.2205)
  line L121 (-9.703, 19.2205) -> (-10.4295, 18.8532)
  line L122 (-10.4295, 18.8532) -> (-10.5946, 19.1797)
  line L123 (-10.5946, 19.1797) -> (-9.8681, 19.547)
  line L124 (-9.8681, 19.547) -> (-10.4326, 20.6632)
  spline S129 degree 2 poles (-10.4326, 20.6632) (-10.5221, 20.8404) (-10.6334, 21.0289) (-10.7186, 21.0907) knots 0 0 0 1 2 2 2
  spline S130 degree 2 poles (-10.7186, 21.0907) (-10.7912, 21.1461) (-10.9877, 21.1389) (-11.1244, 21.0698) knots 0 0 0 1 2 2 2
  spline S131 degree 2 poles (-11.1244, 21.0698) (-11.2206, 21.0212) (-11.3709, 20.8721) (-11.4024, 20.8339) knots 0 0 0 1 2 2 2
  line L125 (-11.4024, 20.8339) -> (-11.4252, 20.8224)
  line L126 (-11.4252, 20.8224) -> (-11.6044, 21.1767)
  spline S132 degree 2 poles (-11.6044, 21.1767) (-11.5084, 21.2634) (-11.2985, 21.414) (-11.1998, 21.4639) knots 0 0 0 1 2 2 2
  line L127 (-12.2822, 17.7236) -> (-12.9603, 21.5248)
  line L128 (-12.9603, 21.5248) -> (-12.5568, 21.7728)
  line L129 (-12.5568, 21.7728) -> (-12.3847, 20.5935)
  line L130 (-12.3847, 20.5935) -> (-10.2644, 18.9636)
  line L131 (-10.2644, 18.9636) -> (-10.6704, 18.7141)
  line L132 (-10.6704, 18.7141) -> (-12.3005, 19.9961)
  line L133 (-12.3005, 19.9961) -> (-11.8907, 17.9642)
  line L134 (-11.8907, 17.9642) -> (-12.2822, 17.7236)
  spline S133 degree 2 poles (-15.9307, 18.2429) (-15.6445, 18.493) (-15.1385, 18.7243) (-14.8866, 18.7938) knots 0 0 0 1 2 2 2
  line L135 (-14.8866, 18.7938) -> (-14.5021, 18.3539)
  line L136 (-14.5021, 18.3539) -> (-14.5277, 18.3315)
  spline S134 degree 2 poles (-14.5277, 18.3315) (-14.8426, 18.3426) (-15.4371, 18.1393) (-15.64, 17.962) knots 0 0 0 1 2 2 2
  spline S135 degree 2 poles (-15.64, 17.962) (-15.9305, 17.7082) (-16.0164, 17.2074) (-15.8428, 17.0088) knots 0 0 0 1 2 2 2
  spline S136 degree 2 poles (-15.8428, 17.0088) (-15.7047, 16.8508) (-15.3771, 16.7906) (-15.1654, 16.8889) knots 0 0 0 1 2 2 2
  spline S137 degree 2 poles (-15.1654, 16.8889) (-15.0138, 16.9611) (-14.7699, 17.0914) (-14.5847, 17.1855) knots 0 0 0 1 2 2 2
  spline S138 degree 2 poles (-14.5847, 17.1855) (-14.4163, 17.2687) (-14.1054, 17.3483) (-13.9456, 17.3335) knots 0 0 0 1 2 2 2
  spline S139 degree 2 poles (-13.9456, 17.3335) (-13.7879, 17.3169) (-13.4929, 17.1603) (-13.3585, 17.0066) knots 0 0 0 1 2 2 2
  spline S140 degree 2 poles (-13.3585, 17.0066) (-13.0785, 16.6862) (-13.1994, 15.8159) (-13.5859, 15.4781) knots 0 0 0 1 2 2 2
  spline S141 degree 2 poles (-13.5859, 15.4781) (-13.808, 15.284) (-14.2775, 15.0281) (-14.519, 14.964) knots 0 0 0 1 2 2 2
  line L137 (-14.519, 14.964) -> (-14.8848, 15.3825)
  line L138 (-14.8848, 15.3825) -> (-14.8592, 15.4049)
  spline S142 degree 2 poles (-14.8592, 15.4049) (-14.6324, 15.3997) (-14.0901, 15.5723) (-13.8744, 15.7608) knots 0 0 0 1 2 2 2
  spline S143 degree 2 poles (-13.8744, 15.7608) (-13.631, 15.9736) (-13.5296, 16.4653) (-13.6919, 16.6511) knots 0 0 0 1 2 2 2